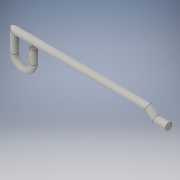
# Autodesk Inventor part: Catch_Lever
Saved by Autodesk Inventor 2016 (Build 200138000, 138)
## iProperties
Created: 2017-11-14
Part Number: Catch_Lever
Material: Generic
Document SubType Name: Modeling
Designer: shen95841
Density: 1 g/cm^3
Appearance: Default
Author: shen95841
Autodesk Inventor part; units mm, degrees
ref_plane "YZ Plane" through (0, 0, 0) normal (1, 0, 0) x (0, 1, 0)
ref_plane "XZ Plane" through (0, 0, 0) normal (0, 1, 0) x (-1, 0, 0)
ref_plane "XY Plane" through (0, 0, 0) normal (0, 0, 1) x (1, 0, 0)
sketch "Sketch1" plane through (0, 0, 0) normal (0, 0, 1) x (1, 0, 0)
  line L0 (0, 0) -> (0, -5.08)
  line L1 (-7.62, 0) -> (-7.62, -5.08)
  arc A0 (-7.62, -5.08) -> (0, -5.08) centre (-3.81, -5.08) ccw
  line L2 (-7.62, 0) -> (-7.62, 2.54)
  line L3 (-7.62, 2.54) -> (45.72, 2.54)
  line L4 (45.72, 2.54) -> (48.7471, 0)
  line L5 (45.72, 2.54) -> (49.6715, 2.54) construction
  line L6 (48.7471, 0) -> (53.8271, 0)
  dimension "d0" = 5.08
  dimension "d1" = 5.08
  dimension "d2" = 7.62
  dimension "d11" = 2.54
  dimension "d13" = 53.34
  dimension "d15" = 2.54
  dimension "d16" = 40
  dimension "d17" = 5.08
  constraints: 14 end point, 3 horizontal, 3 vertical, 2 point on circle, 2 tangent, 1 centre point, 1 equal length
  measures "d0" distance of L0.start L0.end
  measures "d1" distance of L1.start L1.end
  measures "d2" distance between parallel lines of L1 L0
  measures "d11" distance of L1.start L2.end
  measures "d13" distance of L2.end L3.end
  measures "d15" vertical distance of L0.start L3.end
  measures "d16" angle of L4 L5
  measures "d17" distance of L4.end L6.end
sketch "Sketch2" plane through (0, 0, 0) normal (0, 1, 0) x (-1, 0, 0)
  circle A0 centre (0, 0) radius 1.27
  dimension "d10" = 2.54
  constraints: 1 centre point, 1 coincident
  measures "d10" diameter of A0
sweep "Sweep1" add profiles "Sketch2" path "Sketch1" path curves L0 A0 L1 L2 L3 L4 L6
body "Solid1"
